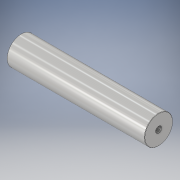
# Autodesk Inventor part: Part2
Saved by Autodesk Inventor 2017 (Build 210142000, 142)
## iProperties
Created: 2017-04-11
Part Number: Part2
Material: Aluminum 6061
Document SubType Name: Modeling
Designer: 193515
Density: 2.7 g/cm^3
Appearance: Aluminum - Polished
Author: 193515
Autodesk Inventor part; units mm, degrees
ref_plane "YZ Plane" through (0, 0, 0) normal (1, 0, 0) x (0, 1, 0)
ref_plane "XZ Plane" through (0, 0, 0) normal (0, 1, 0) x (-1, 0, 0)
ref_plane "XY Plane" through (0, 0, 0) normal (0, 0, 1) x (1, 0, 0)
sketch "Sketch1" plane through (0, 0, 0) normal (1, 0, 0) x (0, 1, 0)
  circle A0 centre (0, 0) radius 11.1125
  dimension "d0" = 22.225
  constraints: 1 centre point, 1 coincident
  measures "d0" diameter of A0
extrude "Extrusion1" add sketch "Sketch1" along normal blind 107.95
chamfer "Chamfer1" distance 0.254 angle 45 1 edges at (107.95, -11.1125, 0)
sketch "Sketch2" plane through (107.95, 0, 0) normal (1, 0, 0) x (0, 0, -1)
  circle A0 centre (0, 0) radius 11.1125 projected
  constraints: 1 coincident
hole "Hole1" at (107.95, 0, 0) direction (-1, 0, 0) diameter 4.9784 depth 22.225 tip angle 118 thread size "1/4-20 UNC" class "2B" standard "ANSI Unified Screw Threads"
body "Solid1"
